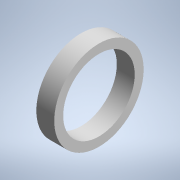
# Autodesk Inventor part: PACK-WSJJ10-8-2
Saved by Autodesk Inventor 2020 (Build 240168000, 168)
## iProperties
Part Number: PACK-WSJJ10-8-2
Material: 一般
Catalog Web Link: www.cadenas.de
Description: PACK-WSJJ,PACK-WSJM-Resin Washer Bulk Packages - Standard
Vendor: MISUMI
Document SubType Name: Modeling
Designer: partserver
Manufacturer: MISUMI
Mass: 0.0565487 g
Surface Area: 1.69646 cm^2
Volume: 0.0565487 cm^3
Density: 1 g/cm^3
Appearance: PSOLRGB-255-255-255
Category: PARTsolutions
Company: MISUMI
PSOL_IDENT_0: {$CADENAS_DATA\23d-libs\misumi\metric\26_washers_collars\pack_wsjj.prj},193 {VTYP=3D},{NB=PACK-WSJJ1
PSOL_IDENT_1: 0-8-2},{LINA=PACK-WSJJ10-8-2},{NN=PACK-WSJJ,PACK-WSJM},{DATE=07.06.2021 03:25:42},{GEOMDATE=02.03.20
PSOL_IDENT_2: 17 08:58:00},{VERSION=},{LINEID=50},{WBVAR=MAT,V,T},{WBNUMERIC=V,T}  {NB=PACK-WSJJ10-8-2},{LINA=PACK
PSOL_IDENT_3: -WSJJ10-8-2},{KT=DUMMY},{PN=PACK-WSJJ10-8-2},{TYPE=PACK-WSJJ},{D=10},{MAT=1},{MATALG='1', 'Polyaceta
PSOL_IDENT_4: l', '2', 'MC Nylon Standard Grade' },{COLOR=White},{COLOR2=1.00,1.00,1.00,0.00},{V=8},{VALG=[3:6/1],
PSOL_IDENT_5: [8]},{T=2},{TALG=[2:3/1],[5]}
NB: PACK-WSJJ10-8-2
NN: PACK-WSJJ,PACK-WSJM
NT: Resin Washer Bulk Packages - Standard
NBSYN: $PN.
LINA: PACK-WSJJ10-8-2
CATALOG: Misumi
PN: PACK-WSJJ10-8-2
D: 10
MAT: Polyacetal
COLOR: White
V: 8
T: 2
SUPPLIER: MISUMI
ARTICLENO: PACK-WSJJ10-8-2
BOMINFO: PACK-WSJJ10-8-2
CREATOR: CADENAS GmbH
Title: PACK-WSJJ10-8-2
Author: Cadenas PARTsolutions
Comments: Resin Washer Bulk Packages - Standard
Autodesk Inventor part; units mm, degrees
ref_plane "YZ Plane" through (0, 0, 0) normal (1, 0, 0) x (0, 1, 0)
ref_plane "XZ Plane" through (0, 0, 0) normal (0, 1, 0) x (-1, 0, 0)
ref_plane "XY Plane" through (0, 0, 0) normal (0, 0, 1) x (1, 0, 0)
sketch "_____1" plane through (0, 0, 0) normal (0, 0, 1) x (1, 0, 0)
  line L0 (1, 0) -> (-1, 0)
  line L1 (-1, 5) -> (-1, 4)
  line L2 (-1, 4) -> (1, 4)
  line L3 (1, 4) -> (1, 5)
  line L4 (1, 5) -> (-1, 5)
  constraints: 10 end point
revolve "Revolution1" add sketch "_____1" angle 360 about axis through (1, 0, 0) along (1, 0, 0)
body "Solid1"
